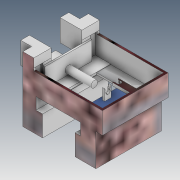
# Autodesk Inventor part: Peça1,61
Saved by Autodesk Inventor 2021 (Build 250183000, 183)
## iProperties
Created: 2020-10-08
Part Number: Peça1,61
Material: Genérico
Document SubType Name: Modeling
Designer: evert
Density: 1 g/cm^3
Appearance: Padrão
Author: evert
Autodesk Inventor part; units mm, degrees
ref_plane "YZ Plane" through (0, 0, 0) normal (1, 0, 0) x (0, 1, 0)
ref_plane "XZ Plane" through (0, 0, 0) normal (0, 1, 0) x (-1, 0, 0)
ref_plane "XY Plane" through (0, 0, 0) normal (0, 0, 1) x (1, 0, 0)
sketch "Esboço2" plane through (0, 0, 0) normal (0, 0, 1) x (1, 0, 0)
  line L0 (0, 0) -> (-5, 0)
  line L1 (-5, 0) -> (-5, -5)
  line L2 (-5, -5) -> (-2, -5)
  line L3 (-2, -5) -> (-2, -15)
  line L4 (-2, -15) -> (-5.6275, -15)
  line L5 (-5.6275, -15) -> (-5.6275, -20)
  line L6 (-5.6275, -20) -> (0, -20)
  line L7 (0, -20) -> (0, -17.5)
  line L8 (0, -17.5) -> (10, -17.5)
  line L9 (10, -17.5) -> (10, -20)
  line L10 (10, -20) -> (15, -20)
  line L11 (15, -20) -> (15, -15)
  line L12 (15, -15) -> (12.5, -15)
  line L13 (12.5, -15) -> (12.5, -5)
  line L14 (12.5, -5) -> (15, -5)
  line L15 (15, 0) -> (15, -5)
  line L16 (15, 0) -> (10, 0)
  line L17 (10, 0) -> (10, -2.5)
  line L18 (10, -2.5) -> (0, -2.5)
  line L19 (0, -2.5) -> (0, 0)
  line L20 (-2.2, -14.8) -> (-2.2, -5.2)
  line L21 (-2.2, -5.2) -> (-4.7, -5.2)
  line L22 (-2.2, -14.8) -> (-4.7, -14.8)
  line L23 (-2.2, -14.8) -> (-5.8275, -14.8)
  line L24 (-5.8275, -14.8) -> (-5.8275, -20)
  line L25 (-5.8275, -20) -> (-5.8275, -20.2)
  line L26 (-5.8275, -20.2) -> (0.2, -20.2)
  line L27 (0.2, -20.2) -> (0.2, -17.7)
  line L28 (0.2, -17.7) -> (9.8, -17.7)
  line L29 (9.8, -17.7) -> (9.8, -18.4636)
  line L30 (9.8, -18.4636) -> (9.8, -20.2)
  line L31 (9.8, -20.2) -> (15.2, -20.2)
  line L32 (15.2, -20.2) -> (15.2, -14.8)
  line L33 (15.2, -14.8) -> (12.7, -14.8)
  line L34 (12.7, -14.8) -> (12.7, -5.2)
  line L35 (12.7, -5.2) -> (15.1265, -5.2)
  line L36 (15.1265, -5.2) -> (15.2, -5.2)
  line L37 (15.2, -5.2) -> (15.2, 0)
  line L38 (-4.7, -5.2) -> (-5.2, -5.2)
  line L39 (-5.2, -5.2) -> (-5.2, 0)
  line L40 (-12.2, 0) -> (-12.2, -24.2)
  line L41 (-12.2, -24.2) -> (22.2, -24.2)
  line L42 (22.2, -24.2) -> (22.2, 0)
  line L43 (15.2, 0) -> (15.2, 0.2)
  line L44 (15.2, 0.2) -> (13.2, 0.2)
  line L45 (22.2, 0) -> (22.2, 1)
  line L46 (22.2, 1) -> (13.2, 1)
  line L47 (13.2, 1) -> (13.2, 0.2)
  line L48 (-12.2, 0) -> (-12.2, 1.2)
  line L49 (-5.2, 0) -> (-5.2, 0.2)
  line L50 (-5.2, 0.2) -> (-3.2, 0.2)
  line L51 (-3.2, 1.2) -> (-12.2, 1.2)
  line L52 (-3.2, 1.2) -> (0, 1.2)
  line L53 (0, 1.2) -> (0, 0.2)
  line L54 (0, 0.2) -> (-3.2, 0.2)
  line L55 (0.5946, -2.5) -> (0.5946, 9.5)
  line L56 (0.5946, 9.5) -> (9.5946, 9.5)
  line L57 (9.5946, 9.5) -> (9.5946, -2.5)
  line L58 (0.5946, -2.5) -> (9.5946, -2.5)
  dimension "d0" = 5
  dimension "d1" = 5
  dimension "d2" = 3
  dimension "d3" = 10
  dimension "d4" = 5
  dimension "d5" = 2.5
  dimension "d6" = 10
  dimension "d7" = 5
  dimension "d8" = 5
  dimension "d9" = 10
  dimension "d11" = 5
  dimension "d12" = 0.2
  dimension "d13" = 0.2
  dimension "d14" = 0.2
  dimension "d15" = 0.2
  dimension "d16" = 0.2
  dimension "d17" = 0.2
  dimension "d19" = 0.2
  dimension "d20" = 0.2
  dimension "d21" = 0.2
  dimension "d22" = 0.2
  dimension "d23" = 0.2
  dimension "d24" = 0.2
  dimension "d25" = 0.2
  dimension "d26" = 0.2
  dimension "d27" = 0.2
  dimension "d28" = 7
  dimension "d29" = 4
  dimension "d30" = 7
  dimension "d31" = 0.2
  dimension "d32" = 2
  dimension "d33" = 1
  dimension "d34" = 0.2
  dimension "d35" = 2
  dimension "d36" = 1
  dimension "d39" = 12
  dimension "d40" = 9
  constraints: 118 end point, 27 perpendicular, 16 point on line, 9 horizontal, 8 vertical, 3 parallel, 1 collinear
  measures "d0" distance of L0.start L0.end
  measures "d1" distance of L0.end L1.end
  measures "d2" distance of L1.end L2.end
  measures "d3" distance of L2.end L3.end
  measures "d4" distance of L4.end L5.end
  measures "d5" distance of L6.end L7.end
  measures "d6" distance of L7.end L8.end
  measures "d7" distance of L9.end L10.end
  measures "d8" distance of L10.end L11.end
  measures "d9" distance of L12.end L13.end
  measures "d11" distance of L15.start L16.end
  measures "d12" distance between parallel lines of L3 L20
  measures "d13" distance between parallel lines of L21 L2
  measures "d14" distance between parallel lines of L4 L22
  measures "d15" distance between parallel lines of L5 L24
  measures "d16" distance between parallel lines of L6 L26
  measures "d17" distance between parallel lines of L7 L27
  measures "d19" distance between parallel lines of L8 L28
  measures "d20" distance between parallel lines of L9 L29
  measures "d21" distance between parallel lines of L31 L10
  measures "d22" distance between parallel lines of L11 L32
  measures "d23" distance between parallel lines of L12 L33
  measures "d24" distance between parallel lines of L34 L13
  measures "d25" distance between parallel lines of L35 L14
  measures "d26" distance between parallel lines of L37 L15
  measures "d27" distance between parallel lines of L1 L39
  measures "d28" distance of L39.end L40.start
  measures "d29" distance from line of L41 L25.end
  measures "d30" distance from line of L42 L31.end
  measures "d31" distance of L37.end L43.end
  measures "d32" distance of L43.end L44.end
  measures "d33" distance of L42.end L45.end
  measures "d34" distance of L39.end L49.end
  measures "d35" distance of L49.end L50.end
  measures "d36" distance between parallel lines of L50 L51
  measures "d39" distance of L55.start L55.end
  measures "d40" distance of L55.end L56.end
extrude "Extrusão1" add sketch "Esboço2" along normal blind 30 contours L22 L23 L24 L25 L26 L27 L28 L29 L30 L31 L32 L33 L34 L35 L36 L37 L43 L44 L47 L46 L45 L42 L41 L40 L48 L51 L52 L53 L54 L50 L49 L39 L38 L21 L20
sketch "Esboço4" plane through (-12.2, -24.2, 0) normal (-1, 0, 0) x (0, 0, 1)
  circle A0 centre (30, 27.7) radius 6 projected
  line L0 (30, 27.7) -> (0, 27.7)
  line L1 (15, 27.7) -> (15, 25.4)
  line L2 (0, 25.4) -> (30, 25.4) projected
  line L3 (0, 27.7) -> (30, 27.7)
  line L4 (30, 27.7) -> (30, 25.4)
  line L5 (30, 25.4) -> (0, 25.4)
  line L6 (0, 25.4) -> (0, 27.7)
  point P0 (0, 24.2)
  constraints: 12 end point, 2 horizontal, 2 midpoint, 2 parallel, 1 perpendicular
extrude "Extrusão2" add sketch "Esboço4" against normal blind 5 contours L0 L4 L2 A0 | A0 L2 L1 L0 | L1 L2 L6 L0 picked at (28.1528, 26.1667)
sketch "Esboço5" plane through (-7.2, -24.2, 0) normal (1, 0, 0) x (0, 0, -1)
  line L0 (-30, 27.7) -> (0, 27.7) projected
  line L1 (0, 27.7) -> (-15, 27.7)
  circle A0 centre (-15, 27.7) radius 1.5
  point P0 (0, 24.2)
  dimension "d48" = 3
  constraints: 2 end point, 1 centre point, 1 coincident, 1 midpoint
  measures "d48" diameter of A0
extrude "Extrusão3" add sketch "Esboço5" along normal blind 13.7
sketch "Esboço6" plane through (-7.2, -24.2, 0) normal (-1, 0, 0) x (0, 0, 1)
  line L0 (13.5, 27.7) -> (16.5, 27.7) projected
  circle A0 centre (15, 27.7) radius 1.5
  point P0 (0, 24.2)
  constraints: 1 centre point, 1 midpoint
extrude "Extrusão4" add sketch "Esboço6" along normal blind 5 contours A0 L0 picked at (15.4855, 27.8197)
sketch "Esboço7" plane through (-12.2, -24.2, 0) normal (-1, 0, 0) x (0, 0, 1)
  circle A0 centre (30, 27.7) radius 6 projected
  line L0 (13.5, 27.7) -> (0, 27.7) projected
  line L1 (30, 33.7) -> (0, 33.7)
  line L2 (0, 33.7) -> (0, 27.7)
  line L3 (0, 27.7) -> (30, 27.7)
  line L4 (30, 27.7) -> (30, 33.7)
  point P0 (0, 24.2)
  constraints: 8 end point, 2 parallel, 1 horizontal, 1 perpendicular, 1 vertical alignment, 1 other
extrude "Extrusão5" add sketch "Esboço7" against normal blind 5 contours L4 L3 A0 | A0 L3 L0 L2 L1 picked at (26.0501, 28.145)
sketch "Esboço8" plane through (-12.2, -24.2, 0) normal (-1, 0, 0) x (0, 0, 1)
  line L0 (30, 33.7) -> (0, 33.7) projected
  line L1 (0, 33.7) -> (0, 35.2)
  line L2 (0, 35.2) -> (30, 35.2)
  line L3 (30, 35.2) -> (30, 33.7)
  line L4 (30, 33.7) -> (0, 33.7)
  line L5 (30, 33.7) -> (30, 25.4) projected
  point P0 (0, 24.2)
  dimension "d55" = 1.5
  constraints: 8 end point, 3 perpendicular, 1 vertical
  measures "d55" distance of L0.end L1.end
extrude "Extrusão6" add sketch "Esboço8" against normal blind 5
sketch "Esboço10" plane through (13.2, 1, 0) normal (0, 1, 0) x (1, 0, 0)
  line L0 (-6.7, -16.5) -> (-6.7, -13.5) projected
  line L1 (-6.7, -15) -> (-6.7, -21.5)
  line L2 (-6.7, -15) -> (-6.7, -8.5)
  line L3 (0, 0) -> (0, -30) projected
  line L4 (0, 0) -> (-13.2, 0)
  line L5 (-3.4, 0) -> (-13, 0) projected
  line L6 (-13.2, 0) -> (-13.2, -8.5)
  line L7 (-13, 0) -> (-13, -30) projected
  line L8 (-13.2, -8.5) -> (0, -8.5)
  line L9 (0, -8.5) -> (0, 0)
  line L10 (2, -30) -> (-3.4, -30) projected
  line L11 (0, -30) -> (0, -21.5)
  line L12 (0, -21.5) -> (-13.2, -21.5)
  line L13 (-13.2, 0) -> (-13.2, -30) projected
  line L14 (-13.2, -21.5) -> (-13.2, -30)
  line L15 (-13.2, -30) -> (0, -30)
  dimension "d58" = 6.5
  dimension "d59" = 6.5
  constraints: 20 end point, 5 perpendicular, 5 point on line, 2 collinear, 1 midpoint, 1 parallel
  measures "d58" distance of L1.start L1.end
  measures "d59" distance of L1.start L2.end
extrude "Extrusão7" add sketch "Esboço10" against normal blind 0.8 contours L12 L3 L10 L15 L7 | L7 L15 L13 L12 | L8 L7 L4 L3 | L8 L6 L4 L7
sketch "Esboço12" plane through (0, 1, 0) normal (0, 1, 0) x (1, 0, 0)
  line L0 (22.2, 0) -> (22.2, -30) projected
  line L1 (22.2, -30) -> (22.2, -15)
  line L2 (13.2, -8.5) -> (13.2, -21.5) projected
  line L3 (13.2, -15) -> (22.2, -15)
  line L4 (13.2, -15) -> (17.7, -15)
  line L5 (13.2, -15) -> (17.7, -15)
  circle A0 centre (17.7, -15) radius 2
  point P0 (0, 0)
  dimension "d62" = 4
  constraints: 8 end point, 3 midpoint, 1 centre point, 1 coincident, 1 collinear, 1 perpendicular
  measures "d62" diameter of A0
extrude "Extrusão8" add sketch "Esboço12" along normal blind 0.5
sketch "Esboço15" plane through (22.2, -24.2, 0) normal (1, 0, 0) x (0, 0, -1)
  line L0 (-30, 25.2) -> (-21.5, 25.2) projected
  line L1 (-30, 25.2) -> (0, 25.2)
  line L2 (0, 25.2) -> (0, 24.2)
  line L3 (0, 24.2) -> (-30, 24.2)
  line L4 (-30, 24.2) -> (-30, 25.2)
  constraints: 8 end point, 2 parallel, 1 horizontal, 1 perpendicular
extrude "Extrusão10" add sketch "Esboço15" along normal blind 3
sketch "Esboço16" plane through (0, 1, 8.5) normal (0, 1, 0) x (1, 0, 0)
  line L0 (22.2, -21.5) -> (25.2, -21.5) projected
  line L1 (25.2, 8.5) -> (23.7, 8.5)
  line L2 (23.7, -21.5) -> (25.2, -21.5)
  line L3 (0, -21.5) -> (25.2, -21.5) projected
  line L4 (-12.2, -21.5) -> (-12.2, 8.5) projected
  line L5 (25.2, -21.5) -> (-12.2, -21.5)
  line L6 (-12.2, -21.5) -> (-12.2, -20.5)
  line L7 (-12.2, -20.5) -> (25.2, -20.5)
  line L8 (25.2, -20.5) -> (25.2, -21.5)
  line L9 (0, 8.5) -> (25.2, 8.5) projected
  line L10 (25.2, 8.5) -> (-12.2, 8.5)
  line L11 (-12.2, 8.5) -> (-12.2, 7.5)
  line L12 (-12.2, 7.5) -> (25.2, 7.5)
  line L13 (25.2, 7.5) -> (25.2, 8.5)
  line L14 (25.2, 8.5) -> (24.2, 8.5)
  line L15 (24.2, 8.5) -> (24.2, -21.5)
  line L16 (24.2, -21.5) -> (25.2, -21.5)
  line L17 (25.2, -21.5) -> (25.2, 8.5)
  point P0 (24.2, 7.5)
  point P1 (24.2, -20.5)
  dimension "d70" = 1
  dimension "d71" = 1
  dimension "d73" = 1
  constraints: 28 end point, 7 parallel, 4 horizontal, 3 perpendicular, 3 point on line, 1 midpoint
  measures "d70" distance between parallel lines of L9 L12
  measures "d71" distance between parallel lines of L7 L3
  measures "d73" distance of L16.end L15.end
extrude "Extrusão11" add sketch "Esboço16" along normal blind 10 contours L3 L5 L4 L7 L15 L0 | L15 L7 L8 L0 | L15 L12 L17 L7 | L15 L1 L13 L12 | L12 L4 L10 L9 L1 L15
sketch "Esboço18" plane through (0, 0, 30) normal (0, 0, 1) x (1, 0, 0)
  line L0 (-12.2, 11) -> (-12.2, -24.2) projected
  line L1 (-12.2, -24.2) -> (22.2, -24.2) projected
  line L2 (-12.2, 11) -> (-11.2, 11)
  line L3 (-11.2, 11) -> (-11.2, -24.2)
  line L4 (-11.2, -24.2) -> (-12.2, -24.2)
  line L5 (-12.2, -24.2) -> (-12.2, 11)
  point P0 (0, 0)
  dimension "d76" = 1
  constraints: 8 end point, 2 parallel, 1 horizontal, 1 perpendicular, 1 point on line
  measures "d76" distance of L3.end L4.end
extrude "Extrusão12" cut sketch "Esboço18" against normal through all
sketch "Esboço20" plane through (0, 1, 8.5) normal (0, 1, 0) x (1, 0, 0)
  line L0 (0, 7.5) -> (0, -20.5) projected
  line L1 (12.7, 8.5) -> (12.7, -21.5) projected
  line L2 (0, 0) -> (12.7, 0)
  line L3 (12.7, 0) -> (12.7, 1)
  line L4 (12.7, 1) -> (0, 1)
  line L5 (0, 1) -> (0, 0)
  line L6 (0, 0) -> (13.2, 0) projected
  line L7 (12.7, 1) -> (13.2, 1)
  line L8 (13.2, 1) -> (13.2, 0)
  line L9 (13.2, 0) -> (12.7, 0)
  line L10 (12.7, 0) -> (12.7, 1)
  line L11 (13.2, 0) -> (13.2, -13) projected
  line L12 (0, -20.5) -> (0, -13) projected
  line L13 (13.2, -13) -> (0, -13)
  line L14 (0, -13) -> (0, -14)
  line L15 (0, -14) -> (13.2, -14)
  line L16 (13.2, -14) -> (13.2, -13)
  point P0 (0, 8.5)
  point P1 (0, -14)
  point P2 (0, -13)
  point P3 (0, 1)
  dimension "d79" = 1
  dimension "d80" = 1
  constraints: 24 end point, 6 parallel, 3 horizontal, 3 perpendicular, 3 point on line
  measures "d79" distance between parallel lines of L4 L2
  measures "d80" distance between parallel lines of L15 L13
extrude "Extrusão13" cut sketch "Esboço20" against normal blind 1 contours L4 L1 L2 L0 | L7 L8 L6 L1 | L13 L1 L15 L0 | L13 L16 L15 L1
sketch "Esboço23" plane through (0, 1, 29) normal (0, 1, 0) x (1, 0, 0)
  line L0 (13.2, 21.5) -> (13.2, 6.5) projected
  line L1 (13.2, 6.5) -> (17.9377, 6.5)
  line L2 (17.9377, 6.5) -> (22.2, 6.5)
  line L3 (22.2, 29) -> (22.2, -1) projected
  line L4 (13.2, 6.5) -> (23.7, 6.5)
  line L5 (13.2, 21.5) -> (0, 21.5) projected
  line L6 (13.2, 21.5) -> (23.7, 21.5)
  line L7 (13.2, 21.5) -> (13.2, 6.5)
  line L8 (23.7, 6.5) -> (23.7, 21.5)
  point P0 (0, 29)
  point P1 (22.2, 21.5)
  point P2 (22.2, 6.5)
  dimension "d91" = 10.5
  constraints: 12 end point, 3 point on line, 2 equal length, 1 horizontal, 1 perpendicular
  measures "d91" distance of L0.end L4.end
extrude "Extrusão16" cut sketch "Esboço23" against normal blind 0.5
sketch "Esboço25" plane through (17.7, 1.5, 15) normal (0, 1, 0) x (1, 0, 0)
  circle A0 centre (0, 0) radius 2 projected
  circle A1 centre (0, 0) radius 2
  circle A2 centre (0, 0) radius 1
  point P0 (-17.7, 15)
  dimension "d96" = 2
  constraints: 3 coincident, 2 centre point
  measures "d96" diameter of A2
extrude "Extrusão17" cut sketch "Esboço25" against normal blind 0.4 contours A0 | A2
sketch "Esboço26" plane through (17.7, 1.1, 15) normal (0, 1, 0) x (1, 0, 0)
  circle A0 centre (0, 0) radius 1
  point P0 (-17.7, 15)
  dimension "d97" = 2
  constraints: 1 centre point
  measures "d97" diameter of A0
extrude "Extrusão18" cut sketch "Esboço26" against normal blind 1.589
sketch "Esboço28" plane through (17.7, 1.1, 15) normal (0, 1, 0) x (1, 0, 0)
  circle A0 centre (0, 0) radius 1 projected
  circle A1 centre (0, 0) radius 2
  point P0 (-17.7, 15)
  constraints: 1 centre point, 1 coincident
extrude "Extrusão19" cut sketch "Esboço28" against normal blind 0.5
sketch "Esboço29" plane through (0, 0.5, 29) normal (0, 1, 0) x (1, 0, 0)
  line L0 (13.2, 6.5) -> (13.2, 21.5) projected
  line L1 (13.2, 21.5) -> (10.2, 21.5)
  line L2 (0, 21.5) -> (23.7, 21.5) projected
  line L3 (10.2, 21.5) -> (10.2, 6.5)
  line L4 (23.7, 6.5) -> (0, 6.5) projected
  line L5 (13.2, 6.5) -> (10.2, 6.5)
  line L6 (10.2, 21.5) -> (13.2, 21.5)
  point P0 (0, 29)
  dimension "d102" = 3
  constraints: 8 end point, 2 perpendicular, 2 point on line, 1 collinear
  measures "d102" distance of L0.end L1.end
extrude "Extrusão20" add sketch "Esboço29" against normal blind 0.5
sketch "Esboço30" plane through (0, 0.5, 29) normal (0, 1, 0) x (1, 0, 0)
  line L0 (6.5, 12.5) -> (6.5, 15.5) projected
  line L1 (6.5, 12.5) -> (6.5, 15.5)
  line L2 (6.5, 15.5) -> (6.5, 12.5)
  line L3 (6.5, 12.5) -> (6.5, 14)
  circle A0 centre (17.7, 14) radius 1 projected
  line L4 (6.5, 14) -> (17.7, 14)
  line L5 (10.2, 6.5) -> (10.2, 21.5) projected
  line L6 (10.2, 14) -> (11.7, 14)
  line L7 (11.7, 14) -> (12.7, 14)
  line L8 (12.7, 29) -> (12.7, -1) projected
  line L9 (11.7, 14) -> (12.7, 14)
  line L10 (11.7, 14) -> (11.7, 15.5)
  line L11 (11.7, 15.5) -> (11.7, 14)
  line L12 (11.7, 14) -> (11.7, 12.5)
  line L13 (11.7, 12.5) -> (12.7, 12.5)
  line L14 (12.7, 12.5) -> (12.7, 15.5)
  line L15 (11.7, 15.5) -> (12.7, 15.5)
  line L16 (12.7, 12.5) -> (12.7, 15.5)
  point P0 (0, 29)
  dimension "d105" = 1.5
  dimension "d106" = 1.5
  dimension "d107" = 1.5
  constraints: 28 end point, 5 collinear, 4 point on line, 3 midpoint, 2 perpendicular, 1 horizontal, 1 vertical
  measures "d105" distance of L6.start L6.end
  measures "d106" distance of L10.end L6.end
  measures "d107" distance of L6.end L12.end
extrude "Extrusão21" add sketch "Esboço30" along normal blind 5 contours L10 L15 L8 L4 | L4 L8 L13 L12
sketch "Esboço32" plane through (12.7, 0.5, 16.5) normal (1, 0, 0) x (0, 0, -1)
  line L0 (3, 0) -> (0, 0) projected
  line L1 (0, 0) -> (0, 1.999)
  line L2 (0, 0) -> (0, 5) projected
  line L3 (0, 1.999) -> (3, 1.999)
  line L4 (3, 0) -> (3, 5) projected
  line L5 (1.5875, 0) -> (1.5, 5)
  line L6 (0, 5) -> (3, 5) projected
  line L7 (1.5525, 1.999) -> (1.535, 2.9988)
  circle A0 centre (1.535, 2.9988) radius 1
  line L8 (3, 0) -> (3, 5) projected
  line L9 (0, 5) -> (0.8269, 3.705)
  line L10 (3, 5) -> (2.2431, 3.705)
  line L11 (0, 5) -> (3, 5)
  point P0 (16.5, -0.5)
  point P1 (1.5175, 1.999)
  point P2 (1.5525, 1.999)
  dimension "d110" = 1.999
  dimension "d111" = 1
  dimension "d112" = 2
  constraints: 14 end point, 5 point on line, 2 point on circle, 1 centre point, 1 coincident, 1 midpoint, 1 perpendicular
  measures "d110" distance of L0.end L1.end
  measures "d111" distance of L7.start L7.end
  measures "d112" diameter of A0
extrude "Extrusão22" cut sketch "Esboço32" against normal blind 1 contours A0 L5 | L5 A0 | L10 A0 L5 L6 | L9 L6 L5 A0
fillet "Arredondamento1" radius 1 2 edges at (12.2, 4.205, 14.2569) (12.2, 4.205, 15.6731)
sketch "Esboço33" plane through (24.2, 1, 1) normal (-1, 0, 0) x (0, 0, 1)
  line L0 (0, 0) -> (14, 0)
  line L1 (14, 0) -> (14, 10)
  line L2 (0, 10) -> (28, 10) projected
  line L3 (14, 10) -> (15.5, 10)
  line L4 (15.5, 10) -> (14, 10)
  line L5 (14, 10) -> (12.5, 10)
  line L6 (12.5, 10) -> (12.5, 7.5)
  line L7 (12.5, 7.5) -> (15.5, 7.5)
  line L8 (15.5, 7.5) -> (15.5, 10)
  point P0 (-1, -1)
  dimension "d117" = 1.5
  dimension "d118" = 1.5
  dimension "d119" = 2.5
  constraints: 16 end point, 2 perpendicular, 2 point on line, 1 collinear, 1 horizontal, 1 midpoint, 1 vertical
  measures "d117" distance of L1.end L3.end
  measures "d118" distance of L1.end L5.end
  measures "d119" distance of L5.end L6.end
extrude "Extrusão23" add sketch "Esboço33" along normal blind 9
sketch "Esboço34" plane through (25.2, 11, 30) normal (0, 1, 0) x (1, 0, 0)
  circle A0 centre (-7.5, 15) radius 1 projected
  line L0 (-10, 16.5) -> (-10, 13.5) projected
  line L1 (-1, 16.5) -> (-10, 16.5) projected
  line L2 (-10, 16.5) -> (-10, 13.5)
  circle A1 centre (-7.5, 15) radius 1
  line L3 (-10, 13.5) -> (-8.0781, 14.184)
  line L4 (-8.0781, 14.184) -> (-8.0781, 15.816)
  line L5 (-10, 13.5) -> (-10, 16.5) projected
  line L6 (-10, 16.5) -> (-8.0781, 15.816)
  point P0 (-25.2, 30)
  dimension "d123" = 2.04
  constraints: 8 end point, 2 point on circle, 1 centre point, 1 coincident, 1 concentric, 1 vertical
  measures "d123" distance of L0.end L3.end
extrude "Extrusão24" cut sketch "Esboço34" against normal blind 2.5
fillet "Arredondamento2" radius 0.2 4 edges at (15.2, 9.75, 16.5) (15.2, 9.75, 13.5) (17.1219, 9.75, 15.816) (17.1219, 9.75, 14.184)
sketch "Esboço38" plane through (-11.2, -24.2, 30) normal (-1, 0, 0) x (0, 0, 1)
  line L0 (0, 35.2) -> (0, 0) projected
  line L1 (-30, 24.2) -> (0, 24.2) projected
  line L2 (0, 24.2) -> (-30, 24.2)
  line L3 (-30, 35.2) -> (0, 35.2) projected
  line L4 (-25, 35.2) -> (-25, 24.2)
  line L5 (-5, 35.2) -> (-5, 24.2)
  line L6 (-5, 24.2) -> (-10, 24.2)
  line L7 (-7.5, 24.2) -> (-22.5, 24.2) projected
  line L8 (-10, 24.2) -> (-10, 27.2)
  line L9 (-10, 27.2) -> (-20, 27.2)
  line L10 (-20, 27.2) -> (-20, 24.2)
  line L11 (-5, 24.2) -> (-5, 29.2)
  line L12 (-5, 29.2) -> (-8, 29.2)
  line L13 (-8, 29.2) -> (-8, 35.2)
  line L14 (-25, 24.2) -> (-25, 29.2)
  line L15 (-25, 29.2) -> (-22, 29.2)
  line L16 (-22, 29.2) -> (-22, 35.2)
  line L17 (-22, 35.2) -> (-8, 35.2)
  point P0 (-5, 24.2)
  dimension "d128" = 20
  dimension "d129" = 5
  dimension "d130" = 5
  dimension "d131" = 3
  dimension "d132" = 10
  dimension "d133" = 5
  dimension "d134" = 3
  dimension "d135" = 3
  constraints: 28 end point, 12 point on line, 7 perpendicular, 2 collinear, 1 vertical
  measures "d128" distance between parallel lines of L5 L4
  measures "d129" distance between parallel lines of L0 L5
  measures "d130" distance of L5.end L6.end
  measures "d131" distance of L6.end L8.end
  measures "d132" distance of L8.end L9.end
  measures "d133" distance of L5.end L11.end
  measures "d134" distance of L11.end L12.end
  measures "d135" distance of L14.end L15.end
extrude "Extrusão25" cut sketch "Esboço38" against normal blind 5 contours L1 L8 L9 L10 L4 L15 L16 L3 L13 L12 L5
sketch "Esboço39" plane through (-7.2, 1.2, 29) normal (0, 1, 0) x (1, 0, 0)
  line L0 (1, 12.5) -> (13.7, 12.5) projected
  line L1 (1, 12.5) -> (1, 4)
  line L2 (1, 4) -> (0, 4) projected
  line L3 (1, 4) -> (0, 4)
  line L4 (1, 24) -> (1, 19) projected
  line L5 (1, 12.5) -> (1, 24)
  line L6 (1, 24) -> (0, 24)
  line L7 (0, 24) -> (0, 24.1)
  line L8 (0, 28) -> (0, 21) projected
  line L9 (0, 24.1) -> (1.1, 24.1)
  line L10 (0, 4) -> (0, 0) projected
  line L11 (0, 4) -> (0, 3.9)
  line L12 (0, 3.9) -> (1.1, 3.9)
  line L13 (1.1, 3.9) -> (1.1, 24.1)
  point P0 (7.2, 29)
  dimension "d138" = 0.1
  dimension "d139" = 1.1
  dimension "d140" = 0.1
  constraints: 18 end point, 3 point on line, 2 collinear, 2 parallel, 2 perpendicular, 1 vertical
  measures "d138" distance of L6.end L7.end
  measures "d139" distance of L7.end L9.end
  measures "d140" distance of L2.end L11.end
extrude "Extrusão26" add sketch "Esboço39" along normal blind 9.8
sketch "Esboço40" plane through (-11.2, 3, 20) normal (0, 1, 0) x (1, 0, 0)
  line L0 (4, 3.5858) -> (4, 0) projected
  line L1 (5, 3.5858) -> (4, 3.5858) projected
  line L2 (4, 0) -> (5, 0)
  line L3 (5, 0) -> (5, 3.5858)
  line L4 (5, 3.5858) -> (4, 3.5858)
  line L5 (4, 3.5858) -> (4, 0)
  line L6 (4, 6.4142) -> (5, 6.4142) projected
  line L7 (4, 6.4142) -> (5, 6.4142)
  line L8 (5, 6.4142) -> (5, 10)
  line L9 (5, 10) -> (4, 10)
  line L10 (4, 10) -> (4, 6.4142)
  point P0 (11.2, 20)
  constraints: 16 end point, 4 parallel, 2 horizontal, 2 perpendicular
extrude "Extrusão27" add sketch "Esboço40" against normal blind 10
sketch "Esboço41" plane through (-7.2, 1.2, 29) normal (0, 1, 0) x (1, 0, 0)
  line L0 (1, 19) -> (1, 15.4142) projected
  line L1 (1, 19) -> (1.8, 19)
  line L2 (1.3725, 29) -> (1.3725, -1) projected
  line L3 (1, 24) -> (1, 4) projected
  line L4 (1, 9.0006) -> (1.8, 9.0006)
  line L5 (1.8, 19) -> (1.8, 9.0006)
  line L6 (1.8, 9.0006) -> (1.8, 3.2006)
  line L7 (1.8, 3.2006) -> (0, 3.2006)
  line L8 (1.8, 19) -> (1.8, 24.8)
  line L9 (1.8, 24.8) -> (0, 24.8)
  line L10 (0, 28) -> (0, 24.1) projected
  line L11 (0, 24.8) -> (0, 24.1)
  line L12 (1.1, 24.1) -> (0, 24.1) projected
  line L13 (0, 24.1) -> (1.1, 24.1)
  line L14 (0, 3.9) -> (0, 0) projected
  line L15 (0, 3.2006) -> (0, 3.9)
  line L16 (0, 3.9) -> (1.1, 3.9) projected
  line L17 (0, 3.9) -> (1.1, 3.9)
  line L18 (1.1, 3.9) -> (1.1, 9.0006)
  line L19 (1.1, 3.9) -> (1.1, 24.1) projected
  line L20 (1.1, 3.9) -> (1.1, 24.1)
  line L21 (0, 28) -> (0, 24.1) projected
  line L22 (0, 24.1) -> (1.1, 24.1)
  line L23 (0, 24.1) -> (0, 24.8)
  point P0 (7.2, 29)
  point P1 (1.1, 19)
  dimension "d149" = 5.8
  dimension "d150" = 5.8
  constraints: 30 end point, 6 perpendicular, 4 collinear, 3 point on line, 3 vertical, 1 horizontal
  measures "d149" distance of L4.end L6.end
  measures "d150" distance of L1.end L8.end
extrude "Extrusão28" add sketch "Esboço41" along normal blind 9.8
sketch "Esboço42" plane through (-7.2, -24.2, 0) normal (1, 0, 0) x (0, 0, -1)
  line L0 (-22, 35.2) -> (-25, 35.2) projected
  line L1 (-22, 35.2) -> (-22, 29.2)
  line L2 (-22, 29.2) -> (-25, 29.1118)
  line L3 (-25, 25.4) -> (-25, 35.2) projected
  line L4 (-25, 35.2) -> (-25, 35.2) projected
  line L5 (-25, 29.2) -> (-22, 29.2) projected
  line L6 (-25, 35.2) -> (-25, 29.2)
  line L7 (-22, 29.2) -> (-22, 35.2) projected
  line L8 (-25, 35.2) -> (-22, 35.2)
  point P0 (0, 24.2)
  constraints: 8 end point, 1 horizontal, 1 perpendicular, 1 point on line
extrude "Extrusão29" add sketch "Esboço42" along normal blind 1.5 contours L1 L5 L3 L0
sketch "Esboço43" plane through (-7.2, -24.2, 0) normal (1, 0, 0) x (0, 0, -1)
  line L0 (-5, 35.2) -> (-5, 35.4) projected
  line L1 (-8, 35.2) -> (-5, 35.2)
  line L2 (-5, 35.2) -> (-8, 35.2) projected
  line L3 (-8, 35.2) -> (-7.9375, 31.75)
  line L4 (-8, 35.2) -> (-8, 29.2086)
  line L5 (-8, 29.2086) -> (-5, 29.2)
  line L6 (-5, 29.2) -> (-5, 35.2)
  point P0 (0, 24.2)
  constraints: 10 end point, 1 collinear, 1 horizontal, 1 vertical
extrude "Extrusão30" add sketch "Esboço43" along normal blind 1.5
sketch "Esboço44" plane through (-11.2, -24.2, 30) normal (-1, 0, 0) x (0, 0, 1)
  line L0 (-7.5, 24.2) -> (-22.5, 24.2) projected
  line L1 (-20, 27.2) -> (-9.9695, 27.2)
  line L2 (-9.9695, 27.2) -> (-9.9695, 24.2)
  line L3 (-9.9695, 24.2) -> (-20, 24.2)
  line L4 (-20, 24.2) -> (-20, 27.2)
  point P0 (-30, 24.2)
  constraints: 8 end point, 2 parallel, 1 horizontal, 1 perpendicular, 1 point on line
extrude "Extrusão31" add sketch "Esboço44" along normal blind 5
sketch "Esboço45" plane through (-11.2, -24.2, 30) normal (-1, 0, 0) x (0, 0, 1)
  line L0 (-8, 35.2) -> (-8, 29.2) projected
  line L1 (-8, 29.2) -> (-8, 39.2)
  line L2 (-8, 39.2) -> (0, 39.2)
  line L3 (-8, 35.2) -> (0, 35.2) projected
  line L4 (0, 39.2) -> (0, 35.2)
  line L5 (0, 35.2) -> (-8, 35.2)
  line L6 (-30, 35.2) -> (-22, 35.2) projected
  line L7 (-22, 35.2) -> (-22, 39.2)
  line L8 (-22, 39.2) -> (-30, 39.2)
  line L9 (-30, 39.2) -> (-30, 35.2)
  line L10 (-8, 29.2) -> (-5, 29.2) projected
  line L11 (-8, 29.2) -> (0, 29.2)
  line L12 (0, 29.2) -> (0, 39.2)
  line L13 (-22, 35.2) -> (-22, 29.2086) projected
  line L14 (-22, 35.2) -> (-22, 29.2086)
  line L15 (-22, 29.2086) -> (-30, 29.2)
  line L16 (-30, 0) -> (-30, 35.2) projected
  line L17 (-30, 39.2) -> (-30, 29.2)
  point P0 (-30, 24.2)
  dimension "d157" = 10
  constraints: 24 end point, 4 collinear, 3 perpendicular, 2 horizontal, 2 point on line, 1 vertical
  measures "d157" distance of L0.end L1.end
extrude "Extrusão32" add sketch "Esboço45" along normal blind 5
sketch "Esboço46" plane through (-11.2, -24.2, 30) normal (1, 0, 0) x (0, 0, -1)
  line L0 (0, 39.2) -> (8, 39.2) projected
  line L1 (8, 39.2) -> (8, 35.2) projected
  line L2 (0, 39.2) -> (8, 39.2)
  line L3 (8, 39.2) -> (8, 35.2)
  line L4 (0, 35.2) -> (0, 39.2) projected
  line L5 (8, 35.2) -> (0, 35.2)
  line L6 (0, 35.2) -> (0, 39.2)
  line L7 (22, 29.2086) -> (22, 39.2) projected
  line L8 (22, 39.2) -> (30, 39.2)
  line L9 (30, 35.2) -> (22, 35.2) projected
  line L10 (30, 39.2) -> (30, 35.2)
  line L11 (30, 35.2) -> (22, 35.2)
  line L12 (22, 35.2) -> (22, 39.2)
  point P0 (30, 24.2)
  constraints: 16 end point, 3 collinear, 3 perpendicular, 2 horizontal
extrude "Extrusão33" add sketch "Esboço46" along normal blind 5
sketch "Esboço47" plane through (-16.2, -24.2, 30) normal (-1, 0, 0) x (0, 0, 1)
  line L0 (0, 29.2) -> (-5, 29.2) projected
  line L1 (-8, 29.2) -> (-5, 29.2)
  line L2 (-8, 29.2) -> (-4, 29.2)
  line L3 (-4, 29.2) -> (-4, 39.2)
  line L4 (0, 39.2) -> (-8, 39.2) projected
  line L5 (0, 39.2) -> (-4, 39.2)
  line L6 (0, 29.2) -> (0, 39.2) projected
  line L7 (0, 39.2) -> (0, 29.2)
  line L8 (0, 29.2) -> (-4, 29.2)
  line L9 (-25, 29.2) -> (-22, 29.2) projected
  line L10 (-22, 29.2) -> (-26, 29.2043)
  line L11 (-22, 29.2086) -> (-30, 29.2) projected
  line L12 (-26, 29.2043) -> (-26, 39.2)
  line L13 (-30, 39.2) -> (-22, 39.2) projected
  line L14 (-30, 39.2) -> (-26, 39.2)
  line L15 (-30, 35.2) -> (-30, 39.2) projected
  line L16 (-30, 39.2) -> (-30, 29.2086)
  line L17 (-30, 29.2086) -> (-26, 29.2043)
  point P0 (-30, 24.2)
  dimension "d163" = 4
  constraints: 22 end point, 5 collinear, 3 midpoint, 3 point on line, 1 perpendicular
  measures "d163" distance of L1.start L2.end
extrude "Extrusão34" cut sketch "Esboço47" against normal blind 5
sketch "Esboço48" plane through (-16.2, 5.0043, 4) normal (0, 0.9999994, 0.0010706) x (1, 0, 0)
  line L0 (5, 4) -> (5, 4.0107) projected
  line L1 (5, 0) -> (5, 4) projected
  line L2 (5, 4.0107) -> (5, 0)
  line L3 (5, 0.0107) -> (0, 0.0107) projected
  line L4 (5, 0) -> (0, 0.0107)
  line L5 (0, 4) -> (5, 4) projected
  line L6 (0.0086, 4.0107) -> (5, 4.0107)
  line L7 (0, 0.0107) -> (0, 0) projected
  line L8 (0, 0) -> (-1.8529, 0)
  line L9 (-1.8529, 0) -> (-1.8529, 4)
  line L10 (-1.8529, 4) -> (0, 4)
  point P0 (16.2, 3.9946)
  constraints: 12 end point, 2 perpendicular, 1 horizontal, 1 vertical, 1 vertical alignment, 2 other
extrude "Extrusão35" cut sketch "Esboço48" against normal blind 5 contours L3 L7 L8 L9 L10 L5 L1
sketch "Esboço50" plane through (22.2, -24.2, 0) normal (0, -1, 0) x (1, 0, 0)
  line L0 (-28.4, 0) -> (-33.4, 0) projected
  line L1 (0, 30) -> (-33.4, 30)
  line L2 (-33.4, 30) -> (-33.4, 0)
  line L3 (-33.4, 0) -> (0, 0)
  line L4 (0, 0) -> (0, 30)
  point P0 (-22.2, 0)
  constraints: 8 end point, 2 parallel, 1 horizontal, 1 perpendicular
extrude "Extrusão36" cut sketch "Esboço50" against normal blind 9.5
sketch "Esboço51" plane through (25.2, 11, 30) normal (0, 1, 0) x (1, 0, 0)
  line L0 (-36.4, 0) -> (-27.4, 0) projected
  line L1 (-31.407, 0) -> (0, 0)
  line L2 (0, 0) -> (0, 30)
  line L3 (0, 30) -> (-31.407, 30)
  line L4 (-31.407, 30) -> (-31.407, 0)
  line L5 (0, 30) -> (-31.407, 30)
  line L6 (-31.407, 30) -> (-31.407, 50)
  line L7 (-31.407, 50) -> (0, 50)
  line L8 (0, 50) -> (0, 30)
  point P0 (-25.2, 30)
  dimension "d172" = 20
  constraints: 16 end point, 4 parallel, 2 horizontal, 2 perpendicular, 2 point on line
  measures "d172" distance of L5.end L6.end
extrude "Extrusão37" cut sketch "Esboço51" against normal blind 1.2 contours L4 L3 L2 L1 L0
